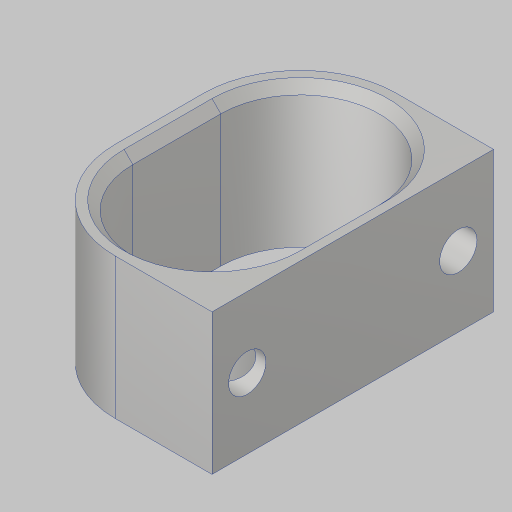
# Autodesk Inventor part: WL-007
Saved by Autodesk Inventor 2023.5 (Build 275446000, 446)
## iProperties
Created: 2025-02-28
Part Number: WL-007
Material: Aluminum 6061
Document SubType Name: Modeling
Designer: slick
Density: 2.7 g/cm^3
Appearance: Aluminum - Flat
Author: slick
Autodesk Inventor part; units mm, degrees
ref_plane "YZ Plane" through (0, 0, 0) normal (1, 0, 0) x (0, 1, 0)
ref_plane "XZ Plane" through (0, 0, 0) normal (0, 1, 0) x (-1, 0, 0)
ref_plane "XY Plane" through (0, 0, 0) normal (0, 0, 1) x (1, 0, 0)
sketch "Sketch1" plane through (0, 0, 0) normal (0, 1, 0) x (-1, 0, 0)
  line L0 (0, -7.9375) -> (0, 7.9375) construction
  line L1 (17.4625, -7.9375) -> (17.4625, 7.9375)
  line L2 (-17.4625, 7.9375) -> (-17.4625, -7.9375)
  arc A0 (-17.4625, -7.9375) -> (17.4625, -7.9375) centre (0, -7.9375) ccw
  arc A1 (17.4625, 7.9375) -> (-17.4625, 7.9375) centre (0, 7.9375) ccw
  line L3 (14.2875, 7.9375) -> (14.2875, -7.9375)
  arc A2 (-14.2875, -7.9375) -> (14.2875, -7.9375) centre (0, -7.9375) ccw
  line L4 (-14.2875, -7.9375) -> (-14.2875, 7.9375)
  arc A3 (14.2875, 7.9375) -> (-14.2875, 7.9375) centre (0, 7.9375) ccw
  point P0 (0, 0)
  point P1 (0, 25.4)
  point P2 (0, -25.4)
  dimension "d1" = 34.925
  dimension "d2" = 3.175
  dimension "d3" = 50.8
  constraints: 12 end point, 10 point on circle, 4 centre point, 4 tangent, 2 parallel, 1 midpoint, 1 vertical, 3 other
  measures "d1" distance between parallel lines of L2 L1
  measures "d2" distance between parallel lines of L1 L3
  measures "d3" distance of point (0, 25.4) point (0, -25.4)
extrude "Extrusion1" add sketch "Sketch1" along normal mid plane 25.4
sketch "Sketch2" plane through (17.4625, -12.7, -7.9375) normal (1, 0, 0) x (0, 0, -1)
  line L0 (0, 0) -> (0, 25.4) construction
  line L1 (-15.875, 25.4) -> (0, 25.4) construction
  line L2 (-15.875, 0) -> (-15.875, 25.4) construction
  line L3 (0, 0) -> (-15.875, 0) construction
  line L4 (-15.875, 0) -> (-15.875, 25.4) construction
  line L5 (-15.875, 25.4) -> (-15.875, 25.4) construction
  line L6 (-15.875, 25.4) -> (-15.875, 0) construction
  line L7 (-15.875, 0) -> (-15.875, 0) construction
  line L8 (0, 0) -> (0, 25.4) construction
  line L9 (0, 25.4) -> (0, 25.4) construction
  line L10 (0, 0) -> (0, 25.4) construction
  line L11 (0, 0) -> (0, 0) construction
  line L12 (-15.875, 25.4) -> (-33.3375, 25.4) construction
  line L13 (17.4625, 0) -> (17.4625, 25.4) construction
  line L14 (-33.3375, 25.4) -> (17.4625, 25.4)
  line L15 (17.4625, 25.4) -> (17.4625, 0)
  line L16 (17.4625, 0) -> (-33.3375, 0)
  line L17 (-33.3375, 0) -> (-33.3375, 25.4)
  line L18 (0, 0) -> (-15.875, 0) construction
  circle A0 centre (-26.9875, 12.7) radius 3.375
  circle A1 centre (11.1125, 12.7) radius 3.375
  line L19 (-26.9875, 12.7) -> (11.1125, 12.7) construction
  point P0 (-7.9375, 12.7)
  point P1 (-7.9375, 12.7)
  dimension "d6" = 6.75
  dimension "d7" = 38.1
  constraints: 10 end point, 2 centre point, 2 horizontal, 2 horizontal alignment, 2 parallel, 1 coincident, 1 collinear, 1 equal radius, 1 midpoint, 1 perpendicular, 1 point on line
  measures "d6" diameter of A0
  measures "d7" distance of L19.start L19.end
extrude "Extrusion2" add sketch "Sketch2" against normal up to next
extrude "Extrusion3" cut sketch "Sketch1" along normal mid plane 25.4 contours L3 A2 L4 A3
chamfer "Chamfer1" distance 1.5875 angle 45 4 edges at (-14.2875, 12.7, 0) (0, 12.7, -22.225) (14.2875, 12.7, 0) (0, 12.7, 22.225)
body "Solid1"
